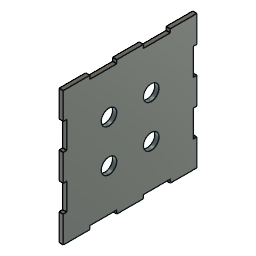
front-and-back-gear-box (Autodesk Fusion 360 design; units mm, degrees)
part number: 2026-06-07-21-52-28-125
Autodesk Fusion 360 part; units mm, degrees
sketch "Sketch1" plane through (0, 0, 0) normal (1, 0, 0) x (0, 1, 0)
  circle A0 centre (65, 125) radius 11
  circle A1 centre (65, 65) radius 11
  circle A2 centre (125, 125) radius 11
  circle A3 centre (125, 65) radius 11
  line L0 (0, 190) -> (38, 190)
  line L1 (38, 190) -> (38, 185)
  line L2 (0, 185) -> (0, 190)
  line L3 (76, 190) -> (76, 185)
  line L4 (76, 185) -> (38, 185)
  line L5 (38, 185) -> (38, 190)
  line L6 (76, 190) -> (114, 190)
  line L7 (114, 190) -> (114, 185)
  line L8 (76, 185) -> (76, 190)
  line L9 (152, 190) -> (152, 185)
  line L10 (152, 185) -> (114, 185)
  line L11 (114, 185) -> (114, 190)
  line L12 (38, 190) -> (0, 190)
  line L13 (190, 190) -> (152, 190)
  line L14 (114, 190) -> (76, 190)
  line L15 (38, 0) -> (0, 0)
  line L16 (38, 5) -> (38, 0)
  line L17 (76, 5) -> (38, 5)
  line L18 (76, 0) -> (76, 5)
  line L19 (114, 0) -> (76, 0)
  line L20 (114, 0) -> (114, 5)
  line L21 (152, 5) -> (114, 5)
  line L22 (190, 0) -> (152, 0)
  line L23 (152, 0) -> (152, 5)
  line L24 (0, 0) -> (38, 0)
  line L25 (76, 0) -> (114, 0)
  line L26 (152, 0) -> (190, 0)
  line L27 (152, 190) -> (190, 190)
  line L28 (152, 185) -> (152, 190)
  line L29 (114, 185) -> (152, 185)
  line L30 (114, 185) -> (114, 190)
  line L31 (76, 190) -> (114, 190)
  line L32 (76, 190) -> (76, 185)
  line L33 (38, 185) -> (76, 185)
  line L34 (0, 190) -> (38, 190)
  line L35 (38, 190) -> (38, 185)
  line L36 (0, 190) -> (5, 190)
  line L37 (5, 152) -> (0, 152)
  line L38 (0, 152) -> (0, 190)
  line L39 (0, 152) -> (5, 152)
  line L40 (5, 152) -> (5, 114)
  line L41 (5, 114) -> (0, 114)
  line L42 (0, 114) -> (5, 114)
  line L43 (5, 76) -> (0, 76)
  line L44 (0, 76) -> (5, 76)
  line L45 (5, 76) -> (5, 38)
  line L46 (5, 38) -> (0, 38)
  line L47 (0, 38) -> (0, 0)
  line L48 (0, 190) -> (0, 152)
  line L49 (0, 190) -> (0, 152)
  line L50 (190, 152) -> (190, 190)
  line L51 (190, 152) -> (185, 152)
  line L52 (185, 152) -> (185, 114)
  line L53 (185, 114) -> (190, 114)
  line L54 (190, 114) -> (190, 76)
  line L55 (185, 76) -> (190, 76)
  line L56 (185, 76) -> (185, 38)
  line L57 (190, 38) -> (190, 0)
  line L58 (190, 152) -> (190, 190)
  line L59 (185, 38) -> (190, 38)
  line L60 (190, 0) -> (190, 38)
  line L61 (190, 76) -> (190, 114)
  line L62 (0, 76) -> (5, 76)
  line L63 (5, 76) -> (5, 38)
  line L64 (5, 38) -> (0, 38)
  line L65 (0, 38) -> (0, 0)
  line L66 (0, 0) -> (38, 0)
  line L67 (38, 5) -> (38, 0)
  line L68 (76, 5) -> (38, 5)
  line L69 (76, 0) -> (76, 5)
  line L70 (114, 0) -> (76, 0)
  line L71 (114, 0) -> (114, 5)
  line L72 (152, 5) -> (114, 5)
  line L73 (152, 0) -> (152, 5)
  line L74 (190, 0) -> (152, 0)
  line L75 (190, 38) -> (190, 0)
  line L76 (185, 38) -> (190, 38)
  line L77 (185, 76) -> (185, 38)
  line L78 (185, 76) -> (190, 76)
  line L79 (190, 76) -> (190, 114)
  line L80 (185, 114) -> (190, 114)
  line L81 (185, 152) -> (185, 114)
  line L82 (190, 152) -> (185, 152)
  line L83 (190, 152) -> (190, 190)
  line L84 (152, 190) -> (190, 190)
  line L85 (152, 185) -> (152, 190)
  line L86 (114, 185) -> (152, 185)
  line L87 (114, 185) -> (114, 190)
  line L88 (76, 190) -> (114, 190)
  line L89 (76, 190) -> (76, 185)
  line L90 (38, 185) -> (76, 185)
  line L91 (38, 190) -> (38, 185)
  line L92 (0, 190) -> (38, 190)
  line L93 (0, 152) -> (0, 190)
  line L94 (0, 152) -> (5, 152)
  line L95 (5, 152) -> (5, 114)
  line L96 (5, 114) -> (0, 114)
  line L97 (0, 114) -> (0, 76)
  line L98 (-0.085, 114.085) -> (-0.085, 75.915)
  line L99 (-0.085, 75.915) -> (4.915, 75.915)
  line L100 (4.915, 75.915) -> (4.915, 38.085)
  line L101 (4.915, 38.085) -> (-0.085, 38.085)
  line L102 (-0.085, 38.085) -> (-0.085, -0.085)
  line L103 (-0.085, -0.085) -> (38.085, -0.085)
  line L104 (38.085, 4.915) -> (38.085, -0.085)
  line L105 (75.915, 4.915) -> (38.085, 4.915)
  line L106 (75.915, -0.085) -> (75.915, 4.915)
  line L107 (114.085, -0.085) -> (75.915, -0.085)
  line L108 (114.085, -0.085) -> (114.085, 4.915)
  line L109 (151.915, 4.915) -> (114.085, 4.915)
  line L110 (151.915, -0.085) -> (151.915, 4.915)
  line L111 (190.085, -0.085) -> (151.915, -0.085)
  line L112 (190.085, 38.085) -> (190.085, -0.085)
  line L113 (185.085, 38.085) -> (190.085, 38.085)
  line L114 (185.085, 75.915) -> (185.085, 38.085)
  line L115 (185.085, 75.915) -> (190.085, 75.915)
  line L116 (190.085, 75.915) -> (190.085, 114.085)
  line L117 (185.085, 114.085) -> (190.085, 114.085)
  line L118 (185.085, 151.915) -> (185.085, 114.085)
  line L119 (190.085, 151.915) -> (185.085, 151.915)
  line L120 (190.085, 151.915) -> (190.085, 190.085)
  line L121 (151.915, 190.085) -> (190.085, 190.085)
  line L122 (151.915, 185.085) -> (151.915, 190.085)
  line L123 (114.085, 185.085) -> (151.915, 185.085)
  line L124 (114.085, 185.085) -> (114.085, 190.085)
  line L125 (75.915, 190.085) -> (114.085, 190.085)
  line L126 (75.915, 190.085) -> (75.915, 185.085)
  line L127 (38.085, 185.085) -> (75.915, 185.085)
  line L128 (38.085, 190.085) -> (38.085, 185.085)
  line L129 (-0.085, 190.085) -> (38.085, 190.085)
  line L130 (-0.085, 151.915) -> (-0.085, 190.085)
  line L131 (-0.085, 151.915) -> (4.915, 151.915)
  line L132 (4.915, 151.915) -> (4.915, 114.085)
  line L133 (4.915, 114.085) -> (-0.085, 114.085)
  circle A4 centre (65, 65) radius 10.915
  circle A5 centre (125, 65) radius 10.915
  circle A6 centre (65, 125) radius 10.915
  circle A7 centre (125, 125) radius 10.915
  dimension "d1" = 190
  dimension "d2" = 190
  dimension "d3" = 22
  dimension "d4" = 22
  dimension "d5" = 22
  dimension "d6" = 22
  dimension "d7" = 60
  dimension "d8" = 60
  dimension "d9" = 60
  dimension "d10" = 65
  dimension "d12" = 65
  dimension "d14" = 65
  dimension "d15" = 38
  dimension "d16" = 5
  dimension "d17" = 38
  dimension "d18" = 5
  dimension "d19" = 38
  dimension "d20" = 38
  dimension "d21" = 5
  dimension "d23" = 5
  dimension "d24" = 38
  dimension "d25" = 5
  dimension "d26" = 38
  dimension "d27" = 5
  dimension "d28" = 38
  dimension "d29" = 5
  dimension "d30" = 38
  dimension "d44" = 0.085
  dimension "d45" = -0.085
  dimension "d46" = -0.085
  dimension "d47" = -0.085
  dimension "d48" = -0.085
  constraint horizontal L24
  constraint vertical L60
  constraint horizontal L13
  constraint vertical L48
  constraint coincident L15.end L24.start
  constraint horizontal L0
  constraint vertical L1
  constraint vertical L2
  constraint vertical L3
  constraint horizontal L4
  constraint vertical L5
  constraint horizontal L6
  constraint vertical L7
  constraint vertical L8
  constraint vertical L9
  constraint horizontal L10
  constraint vertical L11
  constraint collinear L12 L14
  constraint collinear L13 L14
  constraint collinear L24 L25
  constraint collinear L25 L26
  constraint horizontal L36
  constraint horizontal L37
  constraint vertical L38
  constraint horizontal L39
  constraint vertical L40
  constraint horizontal L41
  constraint horizontal L42
  constraint horizontal L43
  constraint horizontal L44
  constraint vertical L45
  constraint horizontal L46
  constraint collinear L58 L61
  constraint collinear L60 L61
  constraint perpendicular L42 L97
  measures "d1" distance of L15.end L22.start
  measures "d2" distance of L15.end L0.start
  measures "d3" diameter of A0
  measures "d4" diameter of A1
  measures "d5" diameter of A2
  measures "d6" diameter of A3
  measures "d7" distance of A0.centre A1.centre
  measures "d8" distance of A2.centre A3.centre
  measures "d9" distance of A0.centre A2.centre
  measures "d10" distance of A2.centre L61
  measures "d12" distance of A1.centre L25
  measures "d14" distance of A3.centre L61
  measures "d15" distance of L0.start L0.end
  measures "d16" distance of L0.start L2.start
  measures "d17" distance of L0.end L3.start
  measures "d18" distance of L0.end L1.end
  measures "d19" distance of L3.start L6.end
  measures "d20" distance of L6.end L9.start
  measures "d21" distance of L6.end L7.end
  measures "d23" distance of L0.start L36.end
  measures "d24" distance of L0.start L37.end
  measures "d25" distance of L37.end L37.start
  measures "d26" distance of L37.end L41.end
  measures "d27" distance of L41.end L40.end
  measures "d28" distance of L41.end L43.end
  measures "d29" distance of L43.end L43.start
  measures "d30" distance of L43.end L46.end
extrude "Extrude1" add sketch "Sketch1" along normal blind 5 contours L0 L1 L2 L3 L4 L5 L6 L7 L8 L9 L10 L11 L12 L13 L14 L15 L16 L17 L18 L19 L20 L21 L22 L23 L24 L25 L26 L27 L28 L29 L30 L31 L32 L33 L34 L35 L36 L37 L38 L39 L40 L41 L42 L43 L44 L45 L46 L47 L48 L49 L50 L51 L52 L53 L54 L55 L56 L57 L58 L59 L60 L61 L62 L63 L64 L65 L66 L67 L68 L69 L70 L71 L72 L73 L74 L75 L76 L77 L78 L79 L80 L81 L82 L83 L84 L85 L86 L87 L88 L89 L90 L91 L92 L93 L94 L95 L96 L97
extrude "Extrude2" add 1 faces at (5, 33.3121, 33.506) along direction (1, 0, 0) blind 1
extrude "Extrude3" add 3 faces at (2, 12.6667, 190) (2, 88.6667, 190) (4, 177.3333, 190) along direction (0, 0, 1) blind 1
extrude "Extrude4" add 3 faces at (4, 190, 165) (2, 190, 101.3333) (4, 190, 25.3333) along direction (0, 1, 0) blind 1
extrude "Extrude5" add 3 faces at (4, 178, 0) (2, 101.3333, 0) (2, 25.3333, 0) along direction (0, 0, -1) blind 1
extrude "Extrude6" add 3 faces at (4, 0, 25) (2, 0, 101.3333) (4, 0, 165) along direction (0, -1, 0) blind 1
extrude "Extrude7" cut 3 faces at (2, 25, -1) (2, 101.3333, -1) (4, 178, -1) along direction (0, 0, 1) blind 1
extrude "Extrude8" cut 3 faces at (4, 191, 25.3333) (2, 191, 101.3333) (4, 191, 165) along direction (0, -1, 0) blind 1
extrude "Extrude9" cut 3 faces at (4, 177.3333, 191) (2, 88.6667, 191) (4, 25, 191) along direction (0, 0, -1) blind 1
extrude "Extrude10" cut 3 faces at (4, -1, 25.3333) (2, -1, 101.3333) (4, -1, 164.6667) along direction (0, 1, 0) blind 1
sketch "Sketch4" plane through (6, 0, 0) normal (1, 0, 0) x (0, 1, 0)
  circle A0 centre (65, 125) radius 11
  circle A1 centre (65, 65) radius 11
  circle A2 centre (125, 125) radius 11
  circle A3 centre (125, 65) radius 11
  line L0 (0, 114) -> (0, 76)
  line L1 (0, 76) -> (5, 76)
  line L2 (5, 76) -> (5, 38)
  line L3 (5, 38) -> (0, 38)
  line L4 (0, 38) -> (0, 0)
  line L5 (0, 0) -> (38, 0)
  line L6 (38, 0) -> (38, 5)
  line L7 (38, 5) -> (76, 5)
  line L8 (76, 5) -> (76, 0)
  line L9 (76, 0) -> (114, 0)
  line L10 (114, 0) -> (114, 5)
  line L11 (114, 5) -> (152, 5)
  line L12 (152, 5) -> (152, 0)
  line L13 (152, 0) -> (190, 0)
  line L14 (190, 0) -> (190, 38)
  line L15 (190, 38) -> (185, 38)
  line L16 (185, 38) -> (185, 76)
  line L17 (185, 76) -> (190, 76)
  line L18 (190, 76) -> (190, 114)
  line L19 (190, 114) -> (185, 114)
  line L20 (185, 114) -> (185, 152)
  line L21 (185, 152) -> (190, 152)
  line L22 (190, 152) -> (190, 190)
  line L23 (190, 190) -> (152, 190)
  line L24 (152, 190) -> (152, 185)
  line L25 (152, 185) -> (114, 185)
  line L26 (114, 185) -> (114, 190)
  line L27 (114, 190) -> (76, 190)
  line L28 (76, 190) -> (76, 185)
  line L29 (76, 185) -> (38, 185)
  line L30 (38, 185) -> (38, 190)
  line L31 (38, 190) -> (0, 190)
  line L32 (0, 190) -> (0, 152)
  line L33 (0, 152) -> (5, 152)
  line L34 (5, 152) -> (5, 114)
  line L35 (5, 114) -> (0, 114)
sketch "Sketch2" plane through (6, 0, 0) normal (1, 0, 0) x (0, 1, 0)
  circle A0 centre (65, 125) radius 11
  circle A1 centre (125, 125) radius 11
  circle A2 centre (125, 65) radius 11
  circle A3 centre (65, 65) radius 11
  line L0 (185, 76) -> (191, 76)
  line L1 (191, 76) -> (191, 114)
  line L2 (191, 114) -> (185, 114)
  line L3 (185, 114) -> (185, 152)
  line L4 (185, 152) -> (191, 152)
  line L5 (191, 152) -> (191, 191)
  line L6 (191, 191) -> (152, 191)
  line L7 (152, 191) -> (152, 185)
  line L8 (152, 185) -> (114, 185)
  line L9 (114, 185) -> (114, 191)
  line L10 (114, 191) -> (76, 191)
  line L11 (76, 191) -> (76, 185)
  line L12 (76, 185) -> (38, 185)
  line L13 (38, 185) -> (38, 191)
  line L14 (38, 191) -> (-1, 191)
  line L15 (-1, 191) -> (-1, 152)
  line L16 (-1, 152) -> (5, 152)
  line L17 (5, 152) -> (5, 114)
  line L18 (5, 114) -> (-1, 114)
  line L19 (-1, 114) -> (-1, 76)
  line L20 (-1, 76) -> (5, 76)
  line L21 (5, 76) -> (5, 38)
  line L22 (5, 38) -> (-1, 38)
  line L23 (-1, 38) -> (-1, -1)
  line L24 (-1, -1) -> (38, -1)
  line L25 (38, -1) -> (38, 5)
  line L26 (38, 5) -> (76, 5)
  line L27 (76, 5) -> (76, -1)
  line L28 (76, -1) -> (114, -1)
  line L29 (114, -1) -> (114, 5)
  line L30 (114, 5) -> (152, 5)
  line L31 (152, 5) -> (152, -1)
  line L32 (152, -1) -> (191, -1)
  line L33 (191, -1) -> (191, 38)
  line L34 (191, 38) -> (185, 38)
  line L35 (185, 38) -> (185, 76)
sketch "Sketch3" plane through (6, 0, 0) normal (1, 0, 0) x (0, 1, 0)
